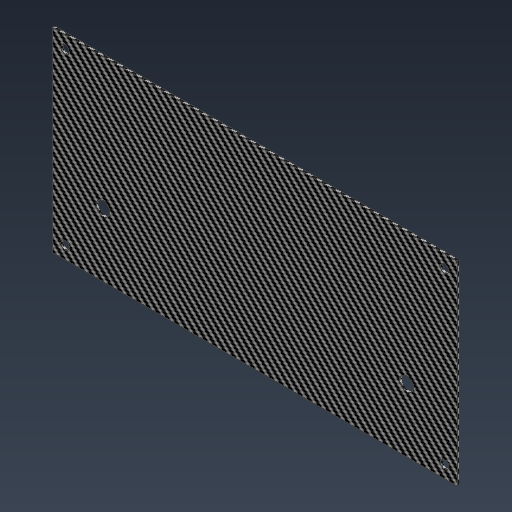
# Autodesk Inventor part: plate4
Saved by Autodesk Inventor 2021 (Build 250183000, 183)
## iProperties
Created: 2021-07-22
Part Number: plate4
Material: CFRP
Document SubType Name: Sheet Metal
Designer: yuta0
Density: 1.43 g/cm^3
Sheet Metal Rule: Default
Appearance: カーボンファイバー
購入先: カーボン
在庫数: 0.0
Author: yuta0
Autodesk Inventor part; units mm, degrees
ref_plane "YZ Plane" through (0, 0, 0) normal (1, 0, 0) x (0, 1, 0)
ref_plane "XZ Plane" through (0, 0, 0) normal (0, 1, 0) x (-1, 0, 0)
ref_plane "XY Plane" through (0, 0, 0) normal (0, 0, 1) x (1, 0, 0)
sketch "スケッチ1" plane through (0, 0, 0) normal (0, 0, 1) x (1, 0, 0)
  line L0 (-80, -38.5) -> (80, -38.5)
  line L1 (80, -38.5) -> (80, 38.5)
  line L2 (80, 38.5) -> (-80, 38.5)
  line L3 (-80, 38.5) -> (-80, -38.5)
  line L4 (-80, -38.5) -> (80, 38.5) construction
  line L5 (80, -38.5) -> (-80, 38.5) construction
  point P0 (0, 0)
  dimension "d0" = 160
  dimension "d1" = 77
  measures "d0" distance of L2.end L1.end
  measures "d1" distance of L1.end L0.end
extrude "プレート1" add sketch "スケッチ1" along normal blind 1
sketch "スケッチ2" plane through (0, 0, 1) normal (0, 0, 1) x (1, 0, 0)
  line L0 (-80, -38.5) -> (-80, 38.5) projected
  line L1 (80, -38.5) -> (-80, -38.5) projected
  line L2 (80, 38.5) -> (80, -38.5) projected
  line L3 (-80, 38.5) -> (80, 38.5) projected
  line L4 (75, 33.5) -> (75, -33.5)
  line L5 (75, -33.5) -> (-75, -33.5)
  line L6 (-75, -33.5) -> (-75, 33.5)
  line L7 (-75, 33.5) -> (75, 33.5)
  point P0 (0, 0)
  dimension "d3" = 5
  constraints: 8 end point, 3 other
  measures "d3" distance between parallel lines of L3 L7
hole "穴1" at (-75, 33.5, 1) at (-75, -33.5, 1) at (75, -33.5, 1) at (75, 33.5, 1) direction (0, 0, -1) diameter 3.4 depth 1 clearance for "Flat Head Machine Screw" size "M3" standard "Ansi Metric M Profile"
sketch "スケッチ3" plane through (0, 0, 1) normal (0, 0, 1) x (1, 0, 0)
  line L0 (80, -38.5) -> (-80, -38.5) projected
  point P0 (0, 0)
  point P1 (-60, -13.5)
  point P2 (60, -13.5)
  dimension "d11" = 60
  dimension "d12" = 60
  dimension "d13" = 25
  dimension "d14" = 25
  measures "d11" horizontal distance of point (0, 0) point (60, -13.5)
  measures "d12" horizontal distance of point (0, 0) point (-60, -13.5)
  measures "d13" distance from line of L0 point (-60, -13.5)
  measures "d14" distance from line of L0 point (60, -13.5)
hole "穴2" at (-60, -13.5, 1) at (60, -13.5, 1) direction (0, 0, -1) diameter 5.5 end through all clearance for "Flat Head Machine Screw" size "M5" standard "Ansi Metric M Profile"
equation "\"d9\" = Thickness"
equation "\"d20\" = Thickness"
equation "\"d2\" = Thickness"
equation "\"BendRadius\" = Thickness"
equation "\"BendReliefWidth\" = Thickness"
equation "\"BendReliefDepth\" = 0.5 * Thickness"
equation "\"CornerReliefSize\" = 4 * Thickness"
equation "\"MinimumRemnant\" = 2 * Thickness"
equation "\"TransitionRadius\" = BendRadius"
equation "\"JacobiRadiusSize\" = Thickness"
equation "\"GapSize\" = Thickness"
equation "\"Thickness\" = 1"
